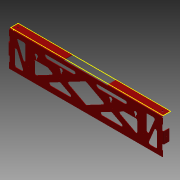
# Autodesk Inventor part: Back
Saved by Autodesk Inventor 2014 (Build 180170000, 170)
## iProperties
Created: 2014-01-06
Part Number: Back
Material: Aluminum 6061
Document SubType Name: Sheet Metal
Designer: Alex
Density: 2.71 g/cm^3
Sheet Metal Rule: Default
Appearance: Red
Author: Alex
Autodesk Inventor part; units mm, degrees
ref_plane "YZ Plane" through (0, 0, 0) normal (1, 0, 0) x (0, 1, 0)
ref_plane "XZ Plane" through (0, 0, 0) normal (0, 1, 0) x (-1, 0, 0)
ref_plane "XY Plane" through (0, 0, 0) normal (0, 0, 1) x (1, 0, 0)
sketch "Sketch1" plane through (0, 0, 0) normal (0, 0, 1) x (1, 0, 0)
  line L0 (-18.5351, 198.7023) -> (673.8689, 198.7023)
  line L1 (673.8689, 198.7023) -> (673.8689, -4.4977)
  line L2 (673.8689, -4.4977) -> (-18.5351, -4.4977)
  line L3 (-18.5351, -4.4977) -> (-18.5351, 198.7023)
  line L4 (-18.5351, 198.7023) -> (-15.9951, 198.7023)
  line L5 (-15.9951, 198.7023) -> (-15.9951, 173.3023)
  line L6 (-15.9951, 173.3023) -> (-18.5351, 173.3023)
  line L7 (-18.5351, 173.3023) -> (-18.5351, 198.7023)
  line L8 (-18.5351, -4.4977) -> (-15.9951, -4.4977)
  line L9 (-15.9951, -4.4977) -> (-15.9951, 20.9023)
  line L10 (-15.9951, 20.9023) -> (-18.5351, 20.9023)
  line L11 (-18.5351, 20.9023) -> (-18.5351, -4.4977)
  line L12 (-18.5351, 71.7023) -> (-15.9951, 71.7023)
  line L13 (-15.9951, 71.7023) -> (-15.9951, 46.3023)
  line L14 (-15.9951, 46.3023) -> (-18.5351, 46.3023)
  line L15 (-18.5351, 46.3023) -> (-18.5351, 71.7023)
  line L16 (-18.5351, 147.9023) -> (-15.9951, 147.9023)
  line L17 (-15.9951, 147.9023) -> (-15.9951, 122.5023)
  line L18 (-15.9951, 122.5023) -> (-18.5351, 122.5023)
  line L19 (-18.5351, 122.5023) -> (-18.5351, 147.9023)
  line L20 (673.8689, 198.7023) -> (671.3289, 198.7023)
  line L21 (671.3289, 198.7023) -> (671.3289, 173.3023)
  line L22 (671.3289, 173.3023) -> (673.8689, 173.3023)
  line L23 (673.8689, 173.3023) -> (673.8689, 198.7023)
  line L24 (673.8689, 147.9023) -> (671.3289, 147.9023)
  line L25 (671.3289, 147.9023) -> (671.3289, 122.5023)
  line L26 (671.3289, 122.5023) -> (673.8689, 122.5023)
  line L27 (673.8689, 122.5023) -> (673.8689, 147.9023)
  line L28 (673.8689, 71.7023) -> (671.3289, 71.7023)
  line L29 (671.3289, 71.7023) -> (671.3289, 46.3023)
  line L30 (671.3289, 46.3023) -> (673.8689, 46.3023)
  line L31 (673.8689, 46.3023) -> (673.8689, 71.7023)
  line L32 (673.8689, 20.9023) -> (671.3289, 20.9023)
  line L33 (671.3289, 20.9023) -> (671.3289, -4.4977)
  line L34 (671.3289, -4.4977) -> (673.8689, -4.4977)
  line L35 (673.8689, -4.4977) -> (673.8689, 20.9023)
  point P0 (0, 0)
  dimension "d0" = 692.404
  dimension "d1" = 203.2
  dimension "d3" = 2.54
  dimension "d4" = 25.4
  dimension "d5" = 2.54
  dimension "d6" = 25.4
  dimension "d7" = 25.4
  dimension "d8" = 25.4
  dimension "d9" = 25.4
  dimension "d10" = 25.4
  dimension "d11" = 2.54
  dimension "d12" = 25.4
  measures "d0" distance of L1.end L2.end
  measures "d1" distance between parallel lines of L2 L0
  measures "d3" distance of L5.end L6.end
  measures "d4" distance of L4.end L5.end
  measures "d5" distance of L10.end L9.end
  measures "d6" distance of L9.end L8.end
  measures "d7" distance of L12.end L13.end
  measures "d8" distance of L16.end L17.end
  measures "d9" distance between parallel lines of L6 L16
  measures "d10" distance between parallel lines of L10 L14
  measures "d11" distance of L22.end L21.end
  measures "d12" distance of L21.end L20.end
extrude "Plate2" add sketch "Sketch1" along normal blind 2.286 contours L0 L21 L22 L1 L24 L25 L26 L28 L29 L30 L32 L33 L2 L9 L10 L3 L14 L13 L12 L18 L17 L16 L6 L5
sketch "Sketch2" plane through (-20.8211, 122.5023, -2.286) normal (-1, 0, 0) x (0, -1, 0)
  line L0 (50.8, 0) -> (0, 0)
  line L1 (0, 0) -> (0, -20.828)
  line L2 (0, -20.828) -> (50.8, -20.828)
  line L3 (50.8, -20.828) -> (50.8, 0)
  constraints: 6 end point, 1 horizontal, 1 perpendicular, 1 vertical
edge flange "Flange1" height 25.4 angle 90 thickness 2.286 bend radius 2.286 thickness toward (-1, 0, 0) relief straight relief width 2.286 relief depth 1.143 corner gap 2.286 corner form 0 edges at (-18.5351, 97.1023, 0) (673.8689, 97.1023, 0) wall of the first edge with corners at (-20.8211, 71.7023, -2.286) (-20.8211, 122.5023, -2.286) (-20.8211, 122.5023, -23.114) (-20.8211, 71.7023, -23.114)
bend "Bend1"
corner "Corner1"
sketch "Sketch4" plane through (0, 0, 2.286) normal (0, 0, 1) x (1, 0, 0)
  line L0 (671.3289, 173.3023) -> (671.3289, 198.7023)
  line L1 (671.3289, 198.7023) -> (-15.9951, 198.7023)
  line L2 (-15.9951, 198.7023) -> (-15.9951, 173.3023)
  line L3 (671.3289, 20.9023) -> (-15.9951, 20.9023)
  line L4 (-15.9951, 20.9023) -> (-15.9951, -4.4977)
  line L5 (-15.9951, -4.4977) -> (671.3289, -4.4977)
  line L6 (671.3289, -4.4977) -> (671.3289, 20.9023)
  line L7 (671.3289, 173.3023) -> (671.3289, 198.7023) projected
  line L8 (-15.9951, 198.7023) -> (-15.9951, 173.3023) projected
  line L9 (-15.9951, 175.5883) -> (671.3289, 175.5883)
  line L10 (-15.9951, 198.7023) -> (671.3289, 198.7023)
  line L11 (671.3289, 198.7023) -> (671.3289, 175.5883)
  line L12 (671.3289, 175.5883) -> (-15.9951, 175.5883)
  line L13 (-15.9951, 175.5883) -> (-15.9951, 198.7023)
  point P0 (0, 0)
  constraints: 24 end point, 5 parallel, 3 perpendicular, 2 horizontal, 2 point on line
extrude "Cut1" cut sketch "Sketch4" against normal blind 2.286
sketch "Sketch12" plane through (671.3289, 177.8743, -2.286) normal (0, 1, 0) x (-1, 0, 0)
  line L0 (687.324, 0) -> (0, 0)
  line L1 (0, 0) -> (0, -33.528)
  line L2 (0, -33.528) -> (687.324, -33.528)
  line L3 (687.324, -33.528) -> (687.324, 0)
  constraints: 6 end point, 1 horizontal, 1 perpendicular, 1 vertical
edge flange "Flange6" height 38.1 angle 90 thickness 2.286 bend radius 2.286 thickness toward (0, 1, 0) relief straight relief width 2.286 relief depth 1.143 edges at (327.6669, 175.5883, 0) wall of the first edge with corners at (-15.9951, 177.8743, -2.286) (671.3289, 177.8743, -2.286) (671.3289, 177.8743, -35.814) (-15.9951, 177.8743, -35.814)
bend "Bend6"
corner "Corner6"
sketch "Sketch15" plane through (0, 0, 2.286) normal (0, 0, 1) x (1, 0, 0)
  line L0 (509.605, 146.3483) -> (446.5777, 113.1433) projected
  arc A0 (440.6581, 113.1433) -> (446.5777, 113.1433) centre (443.6179, 118.7613) ccw projected
  line L1 (440.6581, 113.1433) -> (377.6308, 146.3483) projected
  arc A1 (380.5906, 158.3163) -> (377.6308, 146.3483) centre (380.5906, 151.9663) ccw projected
  line L2 (380.5906, 158.3163) -> (506.6452, 158.3163) projected
  arc A2 (509.605, 146.3483) -> (506.6452, 158.3163) centre (506.6452, 151.9663) ccw projected
  line L3 (214.6757, 81.3153) -> (277.703, 48.1103) projected
  arc A3 (274.7432, 36.1423) -> (277.703, 48.1103) centre (274.7432, 42.4923) ccw projected
  line L4 (274.7432, 36.1423) -> (148.6886, 36.1423) projected
  arc A4 (145.7288, 48.1103) -> (148.6886, 36.1423) centre (148.6886, 42.4923) ccw projected
  line L5 (145.7288, 48.1103) -> (208.7561, 81.3153) projected
  arc A5 (214.6757, 81.3153) -> (208.7561, 81.3153) centre (211.7159, 75.6973) ccw projected
  line L6 (148.6886, 158.3163) -> (274.7432, 158.3163) projected
  arc A6 (277.703, 146.3483) -> (274.7432, 158.3163) centre (274.7432, 151.9663) ccw projected
  line L7 (277.703, 146.3483) -> (214.6757, 113.1433) projected
  arc A7 (208.7561, 113.1433) -> (214.6757, 113.1433) centre (211.7159, 118.7613) ccw projected
  line L8 (208.7561, 113.1433) -> (145.7288, 146.3483) projected
  arc A8 (148.6886, 158.3163) -> (145.7288, 146.3483) centre (148.6886, 151.9663) ccw projected
  line L9 (95.7649, 61.0197) -> (95.7649, 133.4389) projected
  arc A9 (105.0747, 139.0569) -> (95.7649, 133.4389) centre (102.1149, 133.4389) ccw projected
  line L10 (105.0747, 139.0569) -> (173.8051, 102.8473) projected
  arc A10 (173.8051, 91.6113) -> (173.8051, 102.8473) centre (170.8454, 97.2293) ccw projected
  line L11 (173.8051, 91.6113) -> (105.0747, 55.4017) projected
  arc A11 (95.7649, 61.0197) -> (105.0747, 55.4017) centre (102.1149, 61.0197) ccw projected
  line L12 (550.2591, 55.4017) -> (481.5287, 91.6113) projected
  arc A12 (481.5287, 102.8473) -> (481.5287, 91.6113) centre (484.4885, 97.2293) ccw projected
  line L13 (481.5287, 102.8473) -> (550.2591, 139.0569) projected
  arc A13 (559.5689, 133.4389) -> (550.2591, 139.0569) centre (553.2189, 133.4389) ccw projected
  line L14 (559.5689, 133.4389) -> (559.5689, 61.0197) projected
  arc A14 (550.2591, 55.4017) -> (559.5689, 61.0197) centre (553.2189, 61.0197) ccw projected
  line L15 (377.6308, 48.1103) -> (440.6581, 81.3153) projected
  arc A15 (446.5777, 81.3153) -> (440.6581, 81.3153) centre (443.6179, 75.6973) ccw projected
  line L16 (446.5777, 81.3153) -> (509.605, 48.1103) projected
  arc A16 (506.6452, 36.1423) -> (509.605, 48.1103) centre (506.6452, 42.4923) ccw projected
  line L17 (506.6452, 36.1423) -> (380.5906, 36.1423) projected
  arc A17 (377.6308, 48.1103) -> (380.5906, 36.1423) centre (380.5906, 42.4923) ccw projected
  line L18 (405.7071, 91.6113) -> (330.6267, 52.0563) projected
  arc A18 (324.7071, 52.0563) -> (330.6267, 52.0563) centre (327.6669, 57.6743) ccw projected
  line L19 (324.7071, 52.0563) -> (249.6267, 91.6113) projected
  arc A19 (249.6267, 102.8473) -> (249.6267, 91.6113) centre (252.5865, 97.2293) ccw projected
  line L20 (249.6267, 102.8473) -> (324.7071, 142.4023) projected
  arc A20 (330.6267, 142.4023) -> (324.7071, 142.4023) centre (327.6669, 136.7843) ccw projected
  line L21 (330.6267, 142.4023) -> (405.7071, 102.8473) projected
  arc A21 (405.7071, 91.6113) -> (405.7071, 102.8473) centre (402.7474, 97.2293) ccw projected
  line L22 (577.7299, 78.0523) -> (577.7299, 116.1523) projected
  arc A22 (584.0799, 122.5023) -> (577.7299, 116.1523) centre (584.0799, 116.1523) ccw projected
  line L23 (584.0799, 122.5023) -> (622.1799, 122.5023) projected
  arc A23 (628.5299, 116.1523) -> (622.1799, 122.5023) centre (622.1799, 116.1523) ccw projected
  line L24 (628.5299, 116.1523) -> (628.5299, 78.0523) projected
  arc A24 (622.1799, 71.7023) -> (628.5299, 78.0523) centre (622.1799, 78.0523) ccw projected
  line L25 (622.1799, 71.7023) -> (584.0799, 71.7023) projected
  arc A25 (577.7299, 78.0523) -> (584.0799, 71.7023) centre (584.0799, 78.0523) ccw projected
  line L26 (26.8039, 78.0523) -> (26.8039, 116.1523) projected
  arc A26 (33.1539, 122.5023) -> (26.8039, 116.1523) centre (33.1539, 116.1523) ccw projected
  line L27 (33.1539, 122.5023) -> (71.2539, 122.5023) projected
  arc A27 (77.6039, 116.1523) -> (71.2539, 122.5023) centre (71.2539, 116.1523) ccw projected
  line L28 (77.6039, 116.1523) -> (77.6039, 78.0523) projected
  arc A28 (71.2539, 71.7023) -> (77.6039, 78.0523) centre (71.2539, 78.0523) ccw projected
  line L29 (71.2539, 71.7023) -> (33.1539, 71.7023) projected
  arc A29 (26.8039, 78.0523) -> (33.1539, 71.7023) centre (33.1539, 78.0523) ccw projected
  line L30 (584.0799, 46.3023) -> (622.1799, 46.3023) projected
  arc A30 (628.5299, 39.9523) -> (622.1799, 46.3023) centre (622.1799, 39.9523) ccw projected
  line L31 (628.5299, 39.9523) -> (628.5299, 20.9023) projected
  line L32 (671.5829, 20.9023) -> (628.5299, 20.9023) projected
  line L33 (671.5829, 33.6023) -> (671.5829, 20.9023) projected
  line L34 (673.8689, 33.6023) -> (671.5829, 33.6023) projected
  line L35 (673.8689, 59.0023) -> (673.8689, 33.6023) projected
  line L36 (671.5829, 59.0023) -> (673.8689, 59.0023) projected
  line L37 (671.5829, 84.4023) -> (671.5829, 59.0023) projected
  line L38 (673.8689, 84.4023) -> (671.5829, 84.4023) projected
  line L39 (673.8689, 109.8023) -> (673.8689, 84.4023) projected
  line L40 (671.5829, 109.8023) -> (673.8689, 109.8023) projected
  line L41 (671.5829, 135.2023) -> (671.5829, 109.8023) projected
  line L42 (673.8689, 135.2023) -> (671.5829, 135.2023) projected
  line L43 (673.8689, 160.6023) -> (673.8689, 135.2023) projected
  line L44 (671.5829, 160.6023) -> (673.8689, 160.6023) projected
  line L45 (671.5829, 171.0163) -> (671.5829, 160.6023) projected
  line L46 (671.5829, 171.0163) -> (666.5029, 171.0163) projected
  line L47 (666.5029, 171.0163) -> (579.6349, 171.0163) projected
  line L48 (579.6349, 171.0163) -> (574.5549, 171.0163) projected
  line L49 (574.5549, 171.0163) -> (574.5549, 99.3883) projected
  line L50 (574.5549, 99.3883) -> (572.2689, 99.3883) projected
  line L51 (572.2689, 99.3883) -> (572.2689, 171.0163) projected
  line L52 (572.2689, 171.0163) -> (83.0649, 171.0163) projected
  line L53 (83.0649, 171.0163) -> (83.0649, 99.3883) projected
  line L54 (83.0649, 99.3883) -> (80.7789, 99.3883) projected
  line L55 (80.7789, 99.3883) -> (80.7789, 171.0163) projected
  line L56 (80.7789, 171.0163) -> (75.6989, 171.0163) projected
  line L57 (75.6989, 171.0163) -> (-11.1691, 171.0163) projected
  line L58 (-11.1691, 171.0163) -> (-16.2491, 171.0163) projected
  line L59 (-16.2491, 160.6023) -> (-16.2491, 171.0163) projected
  line L60 (-18.5351, 160.6023) -> (-16.2491, 160.6023) projected
  line L61 (-18.5351, 135.2023) -> (-18.5351, 160.6023) projected
  line L62 (-16.2491, 135.2023) -> (-18.5351, 135.2023) projected
  line L63 (-16.2491, 109.8023) -> (-16.2491, 135.2023) projected
  line L64 (-18.5351, 109.8023) -> (-16.2491, 109.8023) projected
  line L65 (-18.5351, 84.4023) -> (-18.5351, 109.8023) projected
  line L66 (-16.2491, 84.4023) -> (-18.5351, 84.4023) projected
  line L67 (-16.2491, 59.0023) -> (-16.2491, 84.4023) projected
  line L68 (-18.5351, 59.0023) -> (-16.2491, 59.0023) projected
  line L69 (-18.5351, 33.6023) -> (-18.5351, 59.0023) projected
  line L70 (-16.2491, 33.6023) -> (-18.5351, 33.6023) projected
  line L71 (-16.2491, 20.9023) -> (-16.2491, 33.6023) projected
  line L72 (26.8039, 20.9023) -> (-16.2491, 20.9023) projected
  line L73 (26.8039, 20.9023) -> (26.8039, 39.9523) projected
  arc A31 (33.1539, 46.3023) -> (26.8039, 39.9523) centre (33.1539, 39.9523) ccw projected
  line L74 (33.1539, 46.3023) -> (71.2539, 46.3023) projected
  arc A32 (77.6039, 39.9523) -> (71.2539, 46.3023) centre (71.2539, 39.9523) ccw projected
  line L75 (77.6039, 39.9523) -> (77.6039, 20.9023) projected
  line L76 (83.0649, 20.9023) -> (77.6039, 20.9023) projected
  line L77 (83.0649, 20.9023) -> (83.0649, 23.4423) projected
  line L78 (83.0649, 23.4423) -> (133.8649, 23.4423) projected
  line L79 (133.8649, 23.4423) -> (133.8649, 20.9023) projected
  line L80 (192.0944, 20.9023) -> (133.8649, 20.9023) projected
  line L81 (192.0944, 20.9023) -> (192.0944, 23.4423) projected
  line L82 (192.0944, 23.4423) -> (242.8944, 23.4423) projected
  line L83 (242.8944, 23.4423) -> (242.8944, 20.9023) projected
  line L84 (301.1239, 20.9023) -> (242.8944, 20.9023) projected
  line L85 (301.1239, 20.9023) -> (301.1239, 23.4423) projected
  line L86 (301.1239, 23.4423) -> (351.9239, 23.4423) projected
  line L87 (351.9239, 23.4423) -> (351.9239, 20.9023) projected
  line L88 (410.1533, 20.9023) -> (351.9239, 20.9023) projected
  line L89 (410.1533, 20.9023) -> (410.1533, 23.4423) projected
  line L90 (410.1533, 23.4423) -> (460.9533, 23.4423) projected
  line L91 (460.9533, 23.4423) -> (460.9533, 20.9023) projected
  line L92 (519.1828, 20.9023) -> (460.9533, 20.9023) projected
  line L93 (519.1828, 20.9023) -> (519.1828, 23.4423) projected
  line L94 (519.1828, 23.4423) -> (569.9828, 23.4423) projected
  line L95 (569.9828, 23.4423) -> (569.9828, 20.9023) projected
  line L96 (577.7299, 20.9023) -> (569.9828, 20.9023) projected
  line L97 (577.7299, 20.9023) -> (577.7299, 39.9523) projected
  arc A33 (584.0799, 46.3023) -> (577.7299, 39.9523) centre (584.0799, 39.9523) ccw projected
  line L98 (-18.5351, 20.9023) -> (673.8689, 20.9023) projected
  line L99 (377.6308, 48.1103) -> (374.6811, 46.5563)
  line L100 (509.605, 48.1103) -> (512.5548, 46.5563)
  line L101 (277.703, 48.1103) -> (280.6528, 46.5563)
  line L102 (145.7288, 48.1103) -> (142.7791, 46.5563)
  line L103 (142.7791, 46.5563) -> (280.6528, 46.5563)
  line L104 (374.6811, 46.5563) -> (512.5548, 46.5563)
  point P0 (0, 0)
  point P1 (373.7342, 46.3023)
  point P2 (513.5016, 46.5563)
  point P3 (281.5996, 46.3023)
  point P4 (141.8322, 46.5563)
  dimension "d139" = 25.654
  dimension "d140" = 25.654
  constraints: 12 end point, 4 tangent, 2 parallel, 2 point on line, 1 other
extrude "Cut5" cut sketch "Sketch15" against normal blind 2.286 contours L0 A0 L1 A1 L2 A2 | L3 A3 L103 A4 L5 A5 | L101 L103 A3 | A4 L103 L102 | L6 A6 L7 A7 L8 A8 | L9 A9 L10 A10 L11 A11 | L12 A12 L13 A13 L14 A14 | L15 A15 L16 A16 L104 A17 | A17 L104 L99 | A16 L100 L104 | L18 A18 L19 A19 L20 A20 L21 A21
fillet "Corner Round1" radius 6.35 4 edges at (512.5548, 46.5563, 1.143) (374.6811, 46.5563, 1.143) (142.7791, 46.5563, 1.143) (280.6528, 46.5563, 1.143)
sketch "Sketch16" plane through (0, 0, 2.286) normal (0, 0, 1) x (1, 0, 0)
  arc A0 (330.6267, 142.4023) -> (324.7071, 142.4023) centre (327.6669, 136.7843) ccw
  line L0 (95.7649, 61.0197) -> (95.7649, 133.4389)
  arc A1 (208.7561, 113.1433) -> (214.6757, 113.1433) centre (211.7159, 118.7613) ccw
  line L1 (559.5689, 133.4389) -> (559.5689, 61.0197)
  line L2 (95.7649, 143.1343) -> (559.5689, 143.1343)
  line L3 (559.5689, 143.1343) -> (559.5689, 112.4113)
  line L4 (559.5689, 112.4113) -> (95.7649, 112.4113)
  line L5 (95.7649, 112.4113) -> (95.7649, 143.1343)
  point P0 (0, 0)
sheet face with bend "Face3" sketch "Sketch16" thickness 2.286 toward (0, 0, -1) bend radius 2.286 relief straight relief width 2.286 relief depth 1.143
bend "Bend7"
fillet "Corner Round2" radius 6.35 10 edges at (151.8294, 143.1343, 1.143) (271.6025, 143.1343, 1.143) (383.7314, 143.1343, 1.143) (503.5045, 143.1343, 1.143) (499.6824, 112.4113, 1.143) (387.5535, 112.4113, 1.143) (267.7804, 112.4113, 1.143) (155.6515, 112.4113, 1.143) (95.7649, 112.4113, 1.143) (559.5689, 112.4113, 1.143)
sketch "Sketch17" plane through (0, 0, 2.286) normal (0, 0, 1) x (1, 0, 0)
  line L0 (270.0321, 143.1343) -> (153.3998, 143.1343) projected
  line L1 (102.1149, 112.4113) -> (154.0811, 112.4113) projected
  line L2 (95.7649, 61.0197) -> (95.7649, 106.0613) projected
  line L3 (107.3218, 137.2034) -> (107.3219, 137.2032)
  line L4 (107.3219, 126.2053) -> (107.3218, 126.2052)
  line L5 (100.972, 126.2052) -> (100.9719, 126.2053)
  line L6 (100.9719, 137.2032) -> (100.972, 137.2034)
  arc A0 (107.3219, 124.7773) -> (100.9719, 124.7773) centre (104.1469, 131.7043) ccw
  line L7 (104.1469, 131.7043) -> (104.1469, 119.0043) construction
  line L8 (100.9719, 124.7773) -> (100.9719, 119.0043)
  line L9 (107.3219, 119.0043) -> (107.3219, 124.7773)
  arc A1 (100.9719, 119.0043) -> (107.3219, 119.0043) centre (104.1469, 119.0043) ccw
  arc A2 (219.0819, 124.7773) -> (212.7319, 124.7773) centre (215.9069, 131.7043) ccw
  line L10 (212.7319, 124.7773) -> (212.7319, 119.0043)
  line L11 (219.0819, 119.0043) -> (219.0819, 124.7773)
  arc A3 (212.7319, 119.0043) -> (219.0819, 119.0043) centre (215.9069, 119.0043) ccw
  arc A4 (330.8419, 124.7773) -> (324.4919, 124.7773) centre (327.6669, 131.7043) ccw
  line L12 (324.4919, 124.7773) -> (324.4919, 119.0043)
  line L13 (330.8419, 119.0043) -> (330.8419, 124.7773)
  arc A5 (324.4919, 119.0043) -> (330.8419, 119.0043) centre (327.6669, 119.0043) ccw
  arc A6 (442.6019, 124.7773) -> (436.2519, 124.7773) centre (439.4269, 131.7043) ccw
  line L14 (436.2519, 124.7773) -> (436.2519, 119.0043)
  line L15 (442.6019, 119.0043) -> (442.6019, 124.7773)
  arc A7 (436.2519, 119.0043) -> (442.6019, 119.0043) centre (439.4269, 119.0043) ccw
  arc A8 (554.3619, 124.7773) -> (548.0119, 124.7773) centre (551.1869, 131.7043) ccw
  line L16 (548.0119, 124.7773) -> (548.0119, 119.0043)
  line L17 (554.3619, 119.0043) -> (554.3619, 124.7773)
  arc A9 (548.0119, 119.0043) -> (554.3619, 119.0043) centre (551.1869, 119.0043) ccw
  point P0 (0, 0)
  point P1 (104.1469, 125.3543)
  point P2 (100.9719, 121.8908)
  point P3 (212.7319, 137.2032)
  point P4 (219.0819, 137.2032)
  point P5 (212.7319, 121.8908)
  point P6 (324.4919, 137.2032)
  point P7 (330.8419, 137.2032)
  point P8 (324.4919, 121.8908)
  point P9 (436.2519, 137.2032)
  point P10 (442.6019, 137.2032)
  point P11 (436.2519, 121.8908)
  point P12 (548.0119, 137.2032)
  point P13 (554.3619, 137.2032)
  point P14 (548.0119, 121.8908)
  dimension "d151" = 15.24
  dimension "d152" = 12.7
  dimension "d153" = 6.35
  dimension "d154" = 11.43
  dimension "d158" = 111.76
  dimension "d163" = 8.382
  constraints: 32 end point, 20 point on circle, 10 centre point, 10 point on line, 2 midpoint, 2 tangent, 1 coincident, 1 horizontal, 1 parallel, 57 other
  measures "d151" diameter of A0
  measures "d152" distance of L7.start L7.end
  measures "d153" diameter of A1
  measures "d154" distance from line of L0 point (104.147, 131.704)
  measures "d158" distance of L7.start A2.centre
  measures "d163" distance from line of point (104.147, 131.704) L2
extrude "Cut6" cut sketch "Sketch17" against normal blind 2.286
sketch "Sketch18" plane through (0, 0, 2.286) normal (0, 0, 1) x (1, 0, 0)
  line L0 (671.3289, 175.5883) -> (-15.9951, 175.5883) projected
  line L1 (-18.5351, 147.9023) -> (-18.5351, 173.3023) projected
  line L2 (-18.5351, 20.9023) -> (673.8689, 20.9023) projected
  line L3 (673.8689, 46.3023) -> (673.8689, 20.9023) projected
  line L4 (6.8649, 156.5383) -> (55.3789, 156.5383)
  line L5 (55.3789, 156.5383) -> (55.3789, 39.9523)
  line L6 (55.3789, 39.9523) -> (6.8649, 39.9523)
  line L7 (6.8649, 39.9523) -> (6.8649, 156.5383)
  line L8 (13.7427, 156.5383) -> (55.3789, 56.4807)
  line L9 (48.5011, 39.9523) -> (6.8649, 140.0099)
  line L10 (648.4689, 156.5383) -> (599.9549, 156.5383)
  line L11 (599.9549, 156.5383) -> (599.9549, 39.9523)
  line L12 (599.9549, 39.9523) -> (648.4689, 39.9523)
  line L13 (648.4689, 39.9523) -> (648.4689, 156.5383)
  line L14 (599.9549, 56.4807) -> (641.5911, 156.5383)
  line L15 (648.4689, 140.0099) -> (606.8327, 39.9523)
  point P0 (-15.9951, 175.5883)
  point P1 (0, 0)
  point P2 (80.7789, 173.3023)
  point P3 (579.1269, 173.3023)
  point P4 (574.5549, 173.3023)
  point P5 (671.3289, 173.3023)
  point P6 (-15.9951, 173.3023)
  dimension "d169" = 19.05
  dimension "d170" = 25.4
  dimension "d171" = 19.05
  dimension "d172" = 25.4
  dimension "d173" = 12.7
  dimension "d174" = 6.35
  dimension "d175" = 6.35
  dimension "d176" = 19.05
  dimension "d177" = 25.4
  dimension "d178" = 19.05
  dimension "d180" = 6.35
  dimension "d181" = 6.35
  dimension "d182" = 12.7
  dimension "d186" = 25.4
  constraints: 24 end point, 8 point on line, 6 parallel, 2 horizontal, 2 perpendicular, 4 other
  measures "d170" distance between parallel lines of L1 L7
  measures "d171" distance between parallel lines of L2 L6
  measures "d172" distance from line of L5 point (80.779, 173.302)
  measures "d173" distance between parallel lines of L9 L8
  measures "d174" distance from line of L4.start L8
  measures "d175" distance from line of L5.end L9
  measures "d176" distance between parallel lines of L2 L12
  measures "d177" distance between parallel lines of L3 L13
  measures "d180" distance from line of L10.start L14
  measures "d181" distance from line of L11.end L15
  measures "d182" distance between parallel lines of L14 L15
  measures "d186" distance from line of point (574.555, 173.302) L11
extrude "Cut7" cut sketch "Sketch18" against normal blind 2.286 contours L4 L5 L8 | L9 L6 L7 | L14 L11 L10 | L13 L12 L15
fillet "Corner Round3" radius 6.35 12 edges at (13.7427, 156.5383, 1.143) (55.3789, 56.4807, 1.143) (48.5011, 39.9523, 1.143) (6.8649, 39.9523, 1.143) (6.8649, 140.0099, 1.143) (55.3789, 156.5383, 1.143) (599.9549, 56.4807, 1.143) (606.8327, 39.9523, 1.143) (648.4689, 39.9523, 1.143) (641.5911, 156.5383, 1.143) (648.4689, 140.0099, 1.143) (599.9549, 156.5383, 1.143)
sketch "Sketch19" plane through (0, 0, 2.286) normal (0, 0, 1) x (1, 0, 0)
  line L0 (-15.9951, 175.5883) -> (-13.4551, 175.5883)
  line L1 (-13.4551, 175.5883) -> (-13.4551, 174.3183)
  line L2 (-13.4551, 174.3183) -> (-15.9951, 174.3183)
  line L3 (-15.9951, 174.3183) -> (-15.9951, 175.5883)
  line L4 (671.3289, 175.5883) -> (668.7889, 175.5883)
  line L5 (668.7889, 175.5883) -> (668.7889, 174.3183)
  line L6 (668.7889, 174.3183) -> (671.3289, 174.3183)
  line L7 (671.3289, 174.3183) -> (671.3289, 175.5883)
  line L8 (-15.9951, 175.5883) -> (-13.4551, 175.5883)
  line L9 (-13.4551, 175.5883) -> (-13.4551, 174.3183)
  line L10 (-13.4551, 174.3183) -> (-15.9951, 174.3183)
  line L11 (-15.9951, 174.3183) -> (-15.9951, 175.5883)
  line L12 (-13.4551, 174.3183) -> (-15.9951, 174.3183)
  line L13 (-15.9951, 174.3183) -> (-15.9951, 175.5883)
  line L14 (-15.9951, 175.5883) -> (-13.4551, 175.5883)
  line L15 (-13.4551, 175.5883) -> (-13.4551, 174.3183)
  point P0 (0, 0)
  dimension "d187" = 2.54
  dimension "d188" = 1.27
  dimension "d189" = 2.54
  dimension "d190" = 1.27
  constraints: 32 end point, 8 parallel, 4 horizontal, 4 perpendicular
  measures "d187" distance of L1.end L2.end
  measures "d188" distance of L0.end L1.end
  measures "d189" distance of L6.end L5.end
  measures "d190" distance of L5.end L4.end
extrude "Cut8" cut sketch "Sketch19" against normal blind 2.286
sketch "Sketch20" plane through (678.4409, 71.7023, -23.114) normal (1, 0, 0) x (0, 0, -1)
  line L0 (-20.828, 50.8) -> (-20.828, 0) projected
  line L1 (0, 50.8) -> (0, 0) projected
  line L2 (-20.828, 50.8) -> (0, 50.8) projected
  circle A0 centre (-10.414, 25.4) radius 1.5875
  circle A1 centre (-10.414, 25.4) radius 1.5875
  point P0 (-23.114, -71.7023)
  dimension "d193" = 3.175
  dimension "d194" = 25.4
  dimension "d195" = 10.414
  dimension "d196" = 10.414
  constraints: 2 centre point, 1 coincident, 1 concentric
  measures "d193" diameter of A0
  measures "d194" distance from line of L2 A0.centre
  measures "d195" distance from line of L1 A0.centre
  measures "d196" distance from line of L0 A0.centre
extrude "Cut9" cut sketch "Sketch20" against normal through all
sketch "Sketch21" plane through (0, 0, 2.286) normal (0, 0, 1) x (1, 0, 0)
  line L0 (500.652, 23.1883) -> (155.4152, 23.1883) projected
  line L1 (155.4152, 44.0163) -> (155.4152, 23.1883) projected
  line L2 (155.4152, 44.0163) -> (500.652, 44.0163) projected
  line L3 (500.652, 44.0163) -> (500.652, 23.1883) projected
  circle A0 centre (206.2152, 33.6023) radius 1.5875
  circle A1 centre (449.852, 33.6023) radius 1.5875
  point P0 (0, 0)
  dimension "d199" = 3.175
  dimension "d200" = 10.414
  dimension "d201" = 10.414
  dimension "d202" = 50.8
  dimension "d203" = 10.414
  dimension "d204" = 50.8
  constraints: 2 centre point
  measures "d199" diameter of A0
  measures "d200" distance from line of L0 A0.centre
  measures "d201" distance from line of L2 A0.centre
  measures "d202" distance from line of L1 A0.centre
  measures "d203" distance from line of L0 A1.centre
  measures "d204" distance from line of L3 A1.centre
extrude "Cut10" cut sketch "Sketch21" against normal blind 2.286 contours A0 | A1
sketch "Sketch22" plane through (0, 0, 2.286) normal (0, 0, 1) x (1, 0, 0)
  circle A0 centre (587.2549, 71.7023) radius 1.5875 projected
  line L0 (576.8409, 122.5023) -> (576.8409, 20.9023) projected
  line L1 (597.6689, 20.9023) -> (576.8409, 20.9023) projected
  line L2 (597.6689, 122.5023) -> (597.6689, 20.9023) projected
  line L3 (576.8409, 122.5023) -> (597.6689, 122.5023) projected
  circle A1 centre (68.0789, 71.7023) radius 1.5875 projected
  line L4 (78.4929, 122.5023) -> (78.4929, 20.9023) projected
  line L5 (57.6649, 20.9023) -> (78.4929, 20.9023) projected
  line L6 (57.6649, 20.9023) -> (57.6649, 122.5023) projected
  line L7 (57.6649, 122.5023) -> (78.4929, 122.5023) projected
  point P0 (0, 0)
extrude "Cut11" cut sketch "Sketch22" against normal blind 2.286 contours A0 | A1
sketch "Sketch23" plane through (-15.9951, 180.1603, -35.814) normal (0, 1, 0) x (1, 0, 0)
  line L0 (0, -33.528) -> (687.324, -33.528) projected
  line L1 (687.324, 0) -> (687.324, -33.528) projected
  line L2 (0, 0) -> (687.324, 0) projected
  line L3 (0, -33.528) -> (0, 0) projected
  point P0 (15.9951, -35.814)
sketch "Sketch24" plane through (-15.9951, 177.8743, -35.814) normal (0, -1, 0) x (1, 0, 0)
  line L0 (2.032, 33.274) -> (2.032, 0.254) projected
  line L1 (35.56, 0.254) -> (2.032, 0.254) projected
  line L2 (35.56, 0.254) -> (35.56, 33.274) projected
  line L3 (35.56, 33.274) -> (2.032, 33.274) projected
  line L4 (685.292, 0.254) -> (685.292, 33.274) projected
  line L5 (651.764, 33.274) -> (685.292, 33.274) projected
  line L6 (651.764, 33.274) -> (651.764, 0.254) projected
  line L7 (651.764, 0.254) -> (685.292, 0.254) projected
  circle A0 centre (668.528, 16.764) radius 3.175
  circle A1 centre (15.9951, 16.764) radius 3.175
  circle A2 centre (668.528, 16.764) radius 3.175 projected
  circle A3 centre (15.9951, 16.764) radius 3.175 projected
  point P0 (15.9951, 35.814)
  dimension "d209" = 6.35
  dimension "d210" = 6.35
  constraints: 2 centre point
  measures "d209" diameter of A0
  measures "d210" diameter of A1
extrude "Cut12" cut sketch "Sketch24" against normal blind 2.286 contours A0 | A1
sketch "Sketch25" plane through (-15.9951, 180.1603, -35.814) normal (0, 1, 0) x (1, 0, 0)
  line L0 (0, 0) -> (687.324, 0) projected
  line L1 (2.54, -35.814) -> (684.784, -35.814) projected
  line L2 (0, -33.528) -> (687.324, -33.528) projected
  line L3 (0, -38.1) -> (0, -33.528) projected
  line L4 (2.54, -38.1) -> (0, -38.1) projected
  line L5 (684.784, -38.1) -> (2.54, -38.1) projected
  line L6 (687.324, -38.1) -> (684.784, -38.1) projected
  line L7 (687.324, -33.528) -> (687.324, -38.1) projected
  line L8 (251.587, 42.672) -> (435.737, 42.672) projected
  line L9 (251.587, -33.528) -> (251.587, 42.672) projected
  line L10 (435.737, -33.528) -> (251.587, -33.528) projected
  line L11 (435.737, 42.672) -> (435.737, -33.528) projected
  line L12 (245.237, 0) -> (442.087, 0)
  line L13 (442.087, 0) -> (442.087, -38.1)
  line L14 (442.087, -38.1) -> (245.237, -38.1)
  line L15 (245.237, -38.1) -> (245.237, 0)
  point P0 (15.9951, -35.814)
  dimension "d213" = 196.85
  dimension "d214" = 6.35
  dimension "d215" = 6.35
  constraints: 8 end point, 2 parallel, 2 point on line, 1 horizontal, 1 perpendicular
  measures "d213" distance of L13.end L14.end
  measures "d214" distance between parallel lines of L11 L13
  measures "d215" distance between parallel lines of L15 L9
extrude "Cut13" cut sketch "Sketch25" against normal blind 4.572 contours L0 L9 L2 L15 | L0 L11 L2 L9 | L2 L13 L1 L15 | L0 L13 L2 L11 | L1 L13 L5 L15
sketch "Sketch26" plane through (0, 0, 2.286) normal (0, 0, 1) x (1, 0, 0)
  arc A0 (330.8419, 124.7773) -> (324.4919, 124.7773) centre (327.6669, 131.7043) ccw
  line L0 (330.8419, 124.7773) -> (330.8419, 119.0043)
  arc A1 (324.4919, 119.0043) -> (330.8419, 119.0043) centre (327.6669, 119.0043) ccw
  line L1 (324.4919, 119.0043) -> (324.4919, 124.7773)
  point P0 (0, 0)
sheet face with bend "Face4" sketch "Sketch26" thickness 2.286 toward (0, 0, -1) bend radius 2.286 relief straight relief width 2.286 relief depth 1.143
bend "Bend8"
sketch "Sketch27" plane through (0, 0, 2.286) normal (0, 0, 1) x (1, 0, 0)
  line L0 (269.3508, 112.4113) -> (385.9831, 112.4113) projected
  arc A0 (388.9428, 111.6794) -> (385.9831, 112.4113) centre (385.9831, 106.0613) ccw projected
  line L1 (388.9428, 111.6794) -> (405.7071, 102.8473) projected
  arc A1 (405.7071, 91.6113) -> (405.7071, 102.8473) centre (402.7474, 97.2293) ccw projected
  line L2 (405.7071, 91.6113) -> (330.6267, 52.0563) projected
  arc A2 (324.7071, 52.0563) -> (330.6267, 52.0563) centre (327.6669, 57.6743) ccw projected
  line L3 (324.7071, 52.0563) -> (249.6267, 91.6113) projected
  arc A3 (249.6267, 102.8473) -> (249.6267, 91.6113) centre (252.5865, 97.2293) ccw projected
  line L4 (249.6267, 102.8473) -> (266.391, 111.6794) projected
  arc A4 (269.3508, 112.4113) -> (266.391, 111.6794) centre (269.3508, 106.0613) ccw projected
  line L5 (509.605, 146.3483) -> (446.5777, 113.1433)
  arc A5 (440.6581, 113.1433) -> (446.5777, 113.1433) centre (443.6179, 118.7613) ccw
  line L6 (440.6581, 113.1433) -> (377.6308, 146.3483)
  arc A6 (380.5906, 158.3163) -> (377.6308, 146.3483) centre (380.5906, 151.9663) ccw
  line L7 (380.5906, 158.3163) -> (506.6452, 158.3163)
  arc A7 (509.605, 146.3483) -> (506.6452, 158.3163) centre (506.6452, 151.9663) ccw
  line L8 (214.6757, 81.3153) -> (277.703, 48.1103)
  arc A8 (274.7432, 36.1423) -> (277.703, 48.1103) centre (274.7432, 42.4923) ccw
  line L9 (274.7432, 36.1423) -> (148.6886, 36.1423)
  arc A9 (145.7288, 48.1103) -> (148.6886, 36.1423) centre (148.6886, 42.4923) ccw
  line L10 (145.7288, 48.1103) -> (208.7561, 81.3153)
  arc A10 (214.6757, 81.3153) -> (208.7561, 81.3153) centre (211.7159, 75.6973) ccw
  line L11 (148.6886, 158.3163) -> (274.7432, 158.3163)
  arc A11 (277.703, 146.3483) -> (274.7432, 158.3163) centre (274.7432, 151.9663) ccw
  line L12 (277.703, 146.3483) -> (214.6757, 113.1433)
  arc A12 (208.7561, 113.1433) -> (214.6757, 113.1433) centre (211.7159, 118.7613) ccw
  line L13 (208.7561, 113.1433) -> (145.7288, 146.3483)
  arc A13 (148.6886, 158.3163) -> (145.7288, 146.3483) centre (148.6886, 151.9663) ccw
  line L14 (95.7649, 61.0197) -> (95.7649, 133.4389)
  arc A14 (105.0747, 139.0569) -> (95.7649, 133.4389) centre (102.1149, 133.4389) ccw
  line L15 (105.0747, 139.0569) -> (173.8051, 102.8473)
  arc A15 (173.8051, 91.6113) -> (173.8051, 102.8473) centre (170.8454, 97.2293) ccw
  line L16 (173.8051, 91.6113) -> (105.0747, 55.4017)
  arc A16 (95.7649, 61.0197) -> (105.0747, 55.4017) centre (102.1149, 61.0197) ccw
  line L17 (550.2591, 55.4017) -> (481.5287, 91.6113)
  arc A17 (481.5287, 102.8473) -> (481.5287, 91.6113) centre (484.4885, 97.2293) ccw
  line L18 (481.5287, 102.8473) -> (550.2591, 139.0569)
  arc A18 (559.5689, 133.4389) -> (550.2591, 139.0569) centre (553.2189, 133.4389) ccw
  line L19 (559.5689, 133.4389) -> (559.5689, 61.0197)
  arc A19 (550.2591, 55.4017) -> (559.5689, 61.0197) centre (553.2189, 61.0197) ccw
  line L20 (377.6308, 48.1103) -> (440.6581, 81.3153)
  arc A20 (446.5777, 81.3153) -> (440.6581, 81.3153) centre (443.6179, 75.6973) ccw
  line L21 (446.5777, 81.3153) -> (509.605, 48.1103)
  arc A21 (506.6452, 36.1423) -> (509.605, 48.1103) centre (506.6452, 42.4923) ccw
  line L22 (506.6452, 36.1423) -> (380.5906, 36.1423)
  arc A22 (377.6308, 48.1103) -> (380.5906, 36.1423) centre (380.5906, 42.4923) ccw
  line L23 (405.7071, 91.6113) -> (330.6267, 52.0563)
  arc A23 (324.7071, 52.0563) -> (330.6267, 52.0563) centre (327.6669, 57.6743) ccw
  line L24 (324.7071, 52.0563) -> (249.6267, 91.6113)
  arc A24 (249.6267, 102.8473) -> (249.6267, 91.6113) centre (252.5865, 97.2293) ccw
  line L25 (249.6267, 102.8473) -> (324.7071, 142.4023)
  arc A25 (330.6267, 142.4023) -> (324.7071, 142.4023) centre (327.6669, 136.7843) ccw
  line L26 (330.6267, 142.4023) -> (405.7071, 102.8473)
  arc A26 (405.7071, 91.6113) -> (405.7071, 102.8473) centre (402.7474, 97.2293) ccw
  line L27 (577.7299, 78.0523) -> (577.7299, 116.1523)
  arc A27 (584.0799, 122.5023) -> (577.7299, 116.1523) centre (584.0799, 116.1523) ccw
  line L28 (584.0799, 122.5023) -> (622.1799, 122.5023)
  arc A28 (628.5299, 116.1523) -> (622.1799, 122.5023) centre (622.1799, 116.1523) ccw
  line L29 (628.5299, 116.1523) -> (628.5299, 78.0523)
  arc A29 (622.1799, 71.7023) -> (628.5299, 78.0523) centre (622.1799, 78.0523) ccw
  line L30 (622.1799, 71.7023) -> (584.0799, 71.7023)
  arc A30 (577.7299, 78.0523) -> (584.0799, 71.7023) centre (584.0799, 78.0523) ccw
  line L31 (26.8039, 78.0523) -> (26.8039, 116.1523)
  arc A31 (33.1539, 122.5023) -> (26.8039, 116.1523) centre (33.1539, 116.1523) ccw
  line L32 (33.1539, 122.5023) -> (71.2539, 122.5023)
  arc A32 (77.6039, 116.1523) -> (71.2539, 122.5023) centre (71.2539, 116.1523) ccw
  line L33 (77.6039, 116.1523) -> (77.6039, 78.0523)
  arc A33 (71.2539, 71.7023) -> (77.6039, 78.0523) centre (71.2539, 78.0523) ccw
  line L34 (71.2539, 71.7023) -> (33.1539, 71.7023)
  arc A34 (26.8039, 78.0523) -> (33.1539, 71.7023) centre (33.1539, 78.0523) ccw
  line L35 (584.0799, 46.3023) -> (622.1799, 46.3023)
  arc A35 (628.5299, 39.9523) -> (622.1799, 46.3023) centre (622.1799, 39.9523) ccw
  line L36 (628.5299, 39.9523) -> (628.5299, 20.9023)
  line L37 (671.5829, 20.9023) -> (628.5299, 20.9023)
  line L38 (671.5829, 33.6023) -> (671.5829, 20.9023)
  line L39 (673.8689, 33.6023) -> (671.5829, 33.6023)
  line L40 (673.8689, 59.0023) -> (673.8689, 33.6023)
  line L41 (671.5829, 59.0023) -> (673.8689, 59.0023)
  line L42 (671.5829, 84.4023) -> (671.5829, 59.0023)
  line L43 (673.8689, 84.4023) -> (671.5829, 84.4023)
  line L44 (673.8689, 109.8023) -> (673.8689, 84.4023)
  line L45 (671.5829, 109.8023) -> (673.8689, 109.8023)
  line L46 (671.5829, 135.2023) -> (671.5829, 109.8023)
  line L47 (673.8689, 135.2023) -> (671.5829, 135.2023)
  line L48 (673.8689, 160.6023) -> (673.8689, 135.2023)
  line L49 (671.5829, 160.6023) -> (673.8689, 160.6023)
  line L50 (671.5829, 171.0163) -> (671.5829, 160.6023)
  line L51 (671.5829, 171.0163) -> (666.5029, 171.0163)
  line L52 (666.5029, 171.0163) -> (579.6349, 171.0163)
  line L53 (579.6349, 171.0163) -> (574.5549, 171.0163)
  line L54 (574.5549, 171.0163) -> (574.5549, 99.3883)
  line L55 (574.5549, 99.3883) -> (572.2689, 99.3883)
  line L56 (572.2689, 99.3883) -> (572.2689, 171.0163)
  line L57 (572.2689, 171.0163) -> (83.0649, 171.0163)
  line L58 (83.0649, 171.0163) -> (83.0649, 99.3883)
  line L59 (83.0649, 99.3883) -> (80.7789, 99.3883)
  line L60 (80.7789, 99.3883) -> (80.7789, 171.0163)
  line L61 (80.7789, 171.0163) -> (75.6989, 171.0163)
  line L62 (75.6989, 171.0163) -> (-11.1691, 171.0163)
  line L63 (-11.1691, 171.0163) -> (-16.2491, 171.0163)
  line L64 (-16.2491, 160.6023) -> (-16.2491, 171.0163)
  line L65 (-18.5351, 160.6023) -> (-16.2491, 160.6023)
  line L66 (-18.5351, 135.2023) -> (-18.5351, 160.6023)
  line L67 (-16.2491, 135.2023) -> (-18.5351, 135.2023)
  line L68 (-16.2491, 109.8023) -> (-16.2491, 135.2023)
  line L69 (-18.5351, 109.8023) -> (-16.2491, 109.8023)
  line L70 (-18.5351, 84.4023) -> (-18.5351, 109.8023)
  line L71 (-16.2491, 84.4023) -> (-18.5351, 84.4023)
  line L72 (-16.2491, 59.0023) -> (-16.2491, 84.4023)
  line L73 (-18.5351, 59.0023) -> (-16.2491, 59.0023)
  line L74 (-18.5351, 33.6023) -> (-18.5351, 59.0023)
  line L75 (-16.2491, 33.6023) -> (-18.5351, 33.6023)
  line L76 (-16.2491, 20.9023) -> (-16.2491, 33.6023)
  line L77 (26.8039, 20.9023) -> (-16.2491, 20.9023)
  line L78 (26.8039, 20.9023) -> (26.8039, 39.9523)
  arc A36 (33.1539, 46.3023) -> (26.8039, 39.9523) centre (33.1539, 39.9523) ccw
  line L79 (33.1539, 46.3023) -> (71.2539, 46.3023)
  arc A37 (77.6039, 39.9523) -> (71.2539, 46.3023) centre (71.2539, 39.9523) ccw
  line L80 (77.6039, 39.9523) -> (77.6039, 20.9023)
  line L81 (83.0649, 20.9023) -> (77.6039, 20.9023)
  line L82 (83.0649, 20.9023) -> (83.0649, 23.4423)
  line L83 (83.0649, 23.4423) -> (133.8649, 23.4423)
  line L84 (133.8649, 23.4423) -> (133.8649, 20.9023)
  line L85 (192.0944, 20.9023) -> (133.8649, 20.9023)
  line L86 (192.0944, 20.9023) -> (192.0944, 23.4423)
  line L87 (192.0944, 23.4423) -> (242.8944, 23.4423)
  line L88 (242.8944, 23.4423) -> (242.8944, 20.9023)
  line L89 (301.1239, 20.9023) -> (242.8944, 20.9023)
  line L90 (301.1239, 20.9023) -> (301.1239, 23.4423)
  line L91 (301.1239, 23.4423) -> (351.9239, 23.4423)
  line L92 (351.9239, 23.4423) -> (351.9239, 20.9023)
  line L93 (410.1533, 20.9023) -> (351.9239, 20.9023)
  line L94 (410.1533, 20.9023) -> (410.1533, 23.4423)
  line L95 (410.1533, 23.4423) -> (460.9533, 23.4423)
  line L96 (460.9533, 23.4423) -> (460.9533, 20.9023)
  line L97 (519.1828, 20.9023) -> (460.9533, 20.9023)
  line L98 (519.1828, 20.9023) -> (519.1828, 23.4423)
  line L99 (519.1828, 23.4423) -> (569.9828, 23.4423)
  line L100 (569.9828, 23.4423) -> (569.9828, 20.9023)
  line L101 (577.7299, 20.9023) -> (569.9828, 20.9023)
  line L102 (577.7299, 20.9023) -> (577.7299, 39.9523)
  arc A38 (584.0799, 46.3023) -> (577.7299, 39.9523) centre (584.0799, 39.9523) ccw
  line L103 (-18.5351, 20.9023) -> (673.8689, 20.9023)
  line L104 (377.6308, 48.1103) -> (374.6811, 46.5563)
  line L105 (509.605, 48.1103) -> (512.5548, 46.5563)
  line L106 (277.703, 48.1103) -> (280.6528, 46.5563)
  line L107 (145.7288, 48.1103) -> (142.7791, 46.5563)
  line L108 (142.7791, 46.5563) -> (280.6528, 46.5563)
  line L109 (374.6811, 46.5563) -> (512.5548, 46.5563)
  point P0 (0, 0)
  point P1 (0, 0)
  point P2 (373.7342, 46.3023)
  point P3 (513.5016, 46.5563)
  point P4 (281.5996, 46.3023)
  point P5 (141.8322, 46.5563)
  dimension "GapSize" = 2.286
  dimension "d223" = 25.654
  dimension "d224" = 25.654
  constraints: 12 end point, 4 tangent, 2 parallel, 2 point on line, 3 other
extrude "Cut14" cut sketch "Sketch27" against normal blind 2.286 contours A4 L25 A25 L26 A0 L0
sketch "Sketch28" plane through (0, 0, 2.286) normal (0, 0, 1) x (1, 0, 0)
  arc A0 (446.5777, 81.3153) -> (440.6581, 81.3153) centre (443.6179, 75.6973) ccw projected
  arc A1 (214.6757, 81.3153) -> (208.7561, 81.3153) centre (211.7159, 75.6973) ccw projected
  arc A2 (212.7319, 119.0043) -> (219.0819, 119.0043) centre (215.9069, 119.0043) ccw projected
  line L0 (419.7419, 198.7023) -> (235.5919, 198.7023) projected
  line L1 (235.5919, 198.7023) -> (235.5919, 20.9023) projected
  line L2 (419.7419, 20.9023) -> (235.5919, 20.9023) projected
  line L3 (419.7419, 198.7023) -> (419.7419, 20.9023) projected
  line L4 (235.5919, 87.8258) -> (197.4919, 87.8258)
  line L5 (197.4919, 87.8258) -> (197.4919, 106.8758)
  line L6 (197.4919, 106.8758) -> (235.5919, 106.8758)
  line L7 (235.5919, 106.8758) -> (235.5919, 87.8258)
  line L8 (419.7419, 106.8758) -> (457.8419, 106.8758)
  line L9 (457.8419, 106.8758) -> (457.8419, 87.8258)
  line L10 (457.8419, 87.8258) -> (419.7419, 87.8258)
  line L11 (419.7419, 87.8258) -> (419.7419, 106.8758)
  circle A3 centre (447.6819, 97.3508) radius 1.5875
  circle A4 centre (207.6519, 97.3508) radius 1.5875
  point P0 (0, 0)
  point P1 (457.8419, 97.3508)
  point P2 (197.4919, 97.3508)
  dimension "d227" = 38.1
  dimension "d228" = 19.05
  dimension "d229" = 12.1285
  dimension "d230" = 12.1285
  dimension "d231" = 38.1
  dimension "d232" = 12.1285
  dimension "d233" = 19.05
  dimension "d234" = 3.175
  dimension "d235" = 10.16
  dimension "d236" = 10.16
  dimension "d237" = 3.175
  constraints: 16 end point, 4 parallel, 2 centre point, 2 horizontal, 2 horizontal alignment, 2 midpoint, 2 perpendicular, 2 point on line
  measures "d227" distance of L5.end L6.end
  measures "d228" distance of L4.end L5.end
  measures "d229" distance from line of A1.centre L4
  measures "d230" distance from line of A2.centre L6
  measures "d231" distance of L9.end L10.end
  measures "d232" distance from line of L10 A0.centre
  measures "d233" distance between parallel lines of L10 L8
  measures "d234" diameter of A3
  measures "d235" distance from line of L9 A3.centre
  measures "d236" distance from line of L5 A4.centre
  measures "d237" diameter of A4
extrude "Cut15" cut sketch "Sketch28" against normal blind 2.286 contours A3 | A4
equation "\"d26\" = Thickness"
equation "\"GapSize\" = Thickness"
equation "\"d14\" = BendReliefWidth"
equation "\"d15\" = BendReliefDepth"
equation "\"d16\" = MinimumRemnant"
equation "\"d17\" = BendRadius"
equation "\"d20\" = BendRadius"
equation "\"d21\" = CornerReliefSize"
equation "\"d22\" = GapSize"
equation "\"d23\" = JacobiRadiusSize"
equation "\"d88\" = BendReliefWidth"
equation "\"d89\" = BendReliefDepth"
equation "\"d90\" = MinimumRemnant"
equation "\"d91\" = BendRadius"
equation "\"d94\" = BendRadius"
equation "\"d95\" = CornerReliefSize"
equation "\"d96\" = GapSize"
equation "\"d97\" = JacobiRadiusSize"
equation "\"BendRadius\" = Thickness"
equation "\"BendReliefWidth\" = Thickness"
equation "\"BendReliefDepth\" = 0.5 * Thickness"
equation "\"CornerReliefSize\" = 4 * Thickness"
equation "\"MinimumRemnant\" = 2 * Thickness"
equation "\"TransitionRadius\" = BendRadius"
equation "\"JacobiRadiusSize\" = BendRadius"
equation "\"d2\" = BendRadius"
equation "\"d13\" = BendRadius"
equation "\"Thickness\" = 2.286"
body "Solid2"
